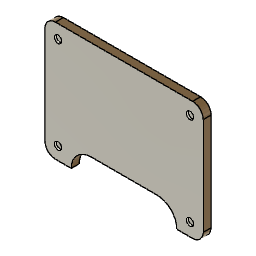
top_access_panel (Autodesk Fusion 360 design; units mm, degrees)
Autodesk Fusion 360 part; units mm, degrees
sketch "Top Access Panel" plane through (0, 0, 0) normal (0, 1, 0) x (1, 0, 0)
  line L0 (0, 0) -> (120, 0)
  line L1 (120, 0) -> (120, -90)
  line L2 (120, -90) -> (0, -90)
  line L3 (0, -90) -> (0, 0)
  dimension "d1" = 120
  dimension "d2" = 90
  constraint horizontal L0
  constraint vertical L1
  constraint horizontal L2
  constraint vertical L3
  constraint coincident L0.start L3.end
  measures "d1" distance of L0.start L0.end
  measures "d2" distance of L0.end L1.end
extrude "Extrude1" add sketch "Top Access Panel" along normal blind 6
fillet "Fillet1" radius 8 4 edges at (0, 3, 90) (120, 3, 90) (120, 3, 0) (0, 3, 0)
sketch "Handle" plane through (0, 6, 0) normal (0, 1, 0) x (-1, 0, 0)
  arc A0 (-8, 0) -> (0, 8) centre (-8, 8) ccw
  line L0 (0, 8) -> (0, 82)
  arc A1 (0, 82) -> (-8, 90) centre (-8, 82) ccw
  line L1 (-8, 90) -> (-112, 90)
  arc A2 (-112, 90) -> (-120, 82) centre (-112, 82) ccw
  line L2 (-120, 82) -> (-120, 8)
  arc A3 (-120, 8) -> (-112, 0) centre (-112, 8) ccw
  line L3 (-112, 0) -> (-8, 0)
  line L4 (-100, 0) -> (-20, 0)
  line L5 (-20, 0) -> (-20, 15)
  line L6 (-20, 15) -> (-100, 15)
  line L7 (-100, 15) -> (-100, 0)
  dimension "d16" = 15
  dimension "d17" = 20
  dimension "d18" = 20
  constraint horizontal L4
  constraint vertical L5
  constraint horizontal L6
  constraint vertical L7
  measures "d16" distance of L4 L6
  measures "d17" distance of L2 L7
  measures "d18" distance of L0 L5
extrude "Extrude3" cut sketch "Handle" against normal blind 6 contours L3 L4 L5 L6 L7
fillet "Fillet2" radius 15 2 edges at (100, 3, 15) (20, 3, 15)
sketch "Sketch4" plane through (0, 0, 0) normal (0, -1, 0) x (1, 0, 0)
  line L0 (35, 15) -> (85, 15)
  arc A0 (100, 0) -> (85, 15) centre (85, 0) ccw
  line L1 (100, 0) -> (112, 0)
  arc A1 (112, 0) -> (120, 8) centre (112, 8) ccw
  line L2 (120, 8) -> (120, 82)
  arc A2 (120, 82) -> (112, 90) centre (112, 82) ccw
  line L3 (112, 90) -> (8, 90)
  arc A3 (8, 90) -> (0, 82) centre (8, 82) ccw
  line L4 (0, 82) -> (0, 8)
  arc A4 (0, 8) -> (8, 0) centre (8, 8) ccw
  line L5 (8, 0) -> (20, 0)
  arc A5 (35, 15) -> (20, 0) centre (35, 0) ccw
  circle A6 centre (10, 79.737) radius 2.75
  circle A7 centre (110, 79.737) radius 2.75
  circle A8 centre (10, 9.737) radius 2.75
  circle A9 centre (110, 9.737) radius 2.75
  dimension "d23" = 5.5
  dimension "d24" = 5.5
  dimension "d25" = 5.5
  dimension "d26" = 5.5
  dimension "d27" = 10
  dimension "d28" = 10
  dimension "d29" = 10
  dimension "d30" = 10
  dimension "d31" = 10.263
  dimension "d32" = 10.263
  dimension "d33" = 9.737
  dimension "d34" = 9.737
  measures "d23" diameter of A6
  measures "d24" diameter of A7
  measures "d25" diameter of A8
  measures "d26" diameter of A9
  measures "d27" distance of L2 A9.centre
  measures "d28" distance of L4 A8.centre
  measures "d29" distance of L4 A6.centre
  measures "d30" distance of L2 A7.centre
  measures "d31" distance of L3 A6.centre
  measures "d32" distance of L3 A7.centre
  measures "d33" distance of L5 A8.centre
  measures "d34" distance of L1 A9.centre
extrude "Extrude4" cut sketch "Sketch4" against normal blind 1.5 contours A6 | A7 | A8 | A9
equation "mdfThickness = 6 mm" comment "Thickness of the MDF fibre board"
equation "d4 = mdfThickness"
equation "filletRadius = 8 mm" comment "Radius to use for fillets"
equation "d15 = filletRadius"
equation "d19 = -mdfThickness"
equation "d27 = 7.5 mm + ( ( 5.5 / 2 ) * 1 mm ) - 0.25 mm"
equation "d28 = 7.5 mm + ( ( 5.5 / 2 ) * 1 mm ) - 0.25 mm"
equation "d29 = 7.5 mm + ( ( 5.5 / 2 ) * 1 mm ) - 0.25 mm"
equation "d30 = 7.5 mm + ( ( 5.5 / 2 ) * 1 mm ) - 0.25 mm"
equation "d31 = 7.763 mm + ( ( 5.5 / 2 ) * 1 mm ) - 0.25 mm"
equation "d32 = 7.763 mm + ( ( 5.5 / 2 ) * 1 mm ) - 0.25 mm"
equation "d33 = 7.237 mm + ( ( 5.5 / 2 ) * 1 mm ) - 0.25 mm"
equation "d34 = 7.237 mm + ( ( 5.5 / 2 ) * 1 mm ) - 0.25 mm"
named bodies: "Top Access Panel"
